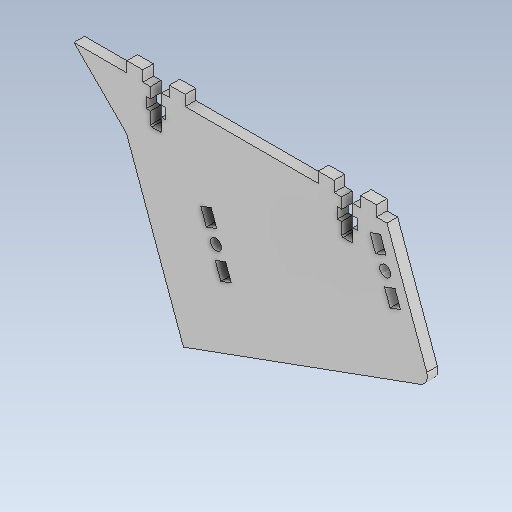
# Autodesk Inventor part: tc_support_front
Saved by Autodesk Inventor 2020.1 (Build 241239000, 239)
## iProperties
Created: 2019-07-16
Part Number: tc_support_front
Material: Acier inoxydable
Document SubType Name: Modeling
Designer: Thibault
Density: 8 g/cm^3
Appearance: Semi-poli
Author: Thibault
Autodesk Inventor part; units mm, degrees
ref_plane "YZ Plane" through (0, 0, 0) normal (1, 0, 0) x (0, 1, 0)
ref_plane "XZ Plane" through (0, 0, 0) normal (0, 1, 0) x (-1, 0, 0)
ref_plane "XY Plane" through (0, 0, 0) normal (0, 0, 1) x (1, 0, 0)
sketch "Anchor (screw side)" plane through (0, 0, 0) normal (0, 0, 1) x (1, 0, 0)
  circle A0 centre (93.7216, 50.3096) radius 1.05
  line L0 (91.2716, 51.3596) -> (88.1716, 51.3596)
  line L1 (88.1716, 51.3596) -> (88.1716, 49.2596)
  line L2 (88.1716, 49.2596) -> (91.2716, 49.2596)
  line L3 (91.2716, 49.2596) -> (91.2716, 51.3596)
  line L4 (99.2716, 51.3596) -> (96.1716, 51.3596)
  line L5 (96.1716, 51.3596) -> (96.1716, 49.2596)
  line L6 (96.1716, 49.2596) -> (99.2716, 49.2596)
  line L7 (99.2716, 49.2596) -> (99.2716, 51.3596)
  line L8 (91.2716, 51.3596) -> (96.1716, 49.2596) construction
  line L9 (96.1716, 51.3596) -> (91.2716, 49.2596) construction
  line L10 (86.1716, 53.3596) -> (101.2716, 53.3596) construction
  line L11 (101.2716, 53.3596) -> (101.2716, 47.2596) construction
  line L12 (101.2716, 47.2596) -> (86.1716, 47.2596) construction
  line L13 (86.1716, 47.2596) -> (86.1716, 53.3596) construction
  point P0 (103.5798, 50.1132)
  dimension "d27" = 2.1
  dimension "d28" = 3.1
  dimension "d29" = 2.1
  dimension "d32" = 4.9
  dimension "d34" = 2
  dimension "d35_1" = 2
  dimension "d36_1" = 2
  dimension "d37" = 2
  measures "d27" diameter of A0
  measures "d28" distance of L2.end L1.end
  measures "d29" distance of L1.end L0.end
  measures "d32" distance between parallel lines of L5 L3
  measures "d34" distance between parallel lines of L0 L10
  measures "d35_1" distance between parallel lines of L12 L2
  measures "d36_1" distance between parallel lines of L11 L7
  measures "d37" distance between parallel lines of L13 L1
sketch "Anchor (nut side)" plane through (0, 0, 0) normal (0, 0, 1) x (1, 0, 0)
  line L0 (10, 0) -> (8.55, 0)
  line L1 (8.55, 0) -> (8.55, -2)
  line L2 (8.55, -2) -> (9.35, -2)
  line L3 (9.35, -2) -> (9.35, -4)
  line L4 (5.65, -4) -> (5.65, -2)
  line L5 (5.65, -2) -> (6.45, -2)
  line L6 (6.45, -2) -> (6.45, 0)
  line L7 (6.45, 0) -> (5, 0)
  line L8 (2, 0) -> (2, 2)
  line L9 (2, 0) -> (3, 0) construction
  line L10 (2, 2) -> (5, 2)
  line L11 (5, 2) -> (5, 0)
  line L12 (10, 0) -> (10, 2)
  line L13 (10, 2) -> (13, 2)
  line L14 (13, 2) -> (13, 0)
  line L15 (0, 0) -> (2, 0)
  line L16 (13, 0) -> (15, 0)
  line L17 (5.65, -4) -> (6.45, -4)
  line L18 (9.35, -4) -> (8.55, -4)
  line L19 (6.45, -4) -> (6.45, -6.25)
  line L20 (8.55, -4) -> (8.55, -6.25)
  line L21 (6.7, -6.5) -> (7.5, -6.5)
  arc A0 (6.45, -6.25) -> (6.7, -6.5) centre (6.7, -6.25) ccw
  arc A1 (8.3, -6.5) -> (8.55, -6.25) centre (8.3, -6.25) ccw
  line L22 (7.5, -6.5) -> (8.3, -6.5)
  line L23 (7.5, -3.8983) -> (7.5, -9.959) construction
  point P0 (9.1321, -0.6227)
  point P1 (6.45, -6.5)
  point P2 (8.55, -6.5)
  dimension "d3" = 2
  dimension "d7" = 5
  dimension "d10" = 1.45
  dimension "d11" = 2
  dimension "d12" = 0.8
  dimension "d13" = 2
  dimension "d14" = 0.8
  dimension "d15" = 2.1
  dimension "d18" = 2
  dimension "d19" = 0.8
  dimension "d20" = 0.8
  dimension "d21" = 2.5
  dimension "d22" = 2.5
  dimension "d23" = 2.1
  dimension "d38" = 2
  dimension "d39" = 0.25
  dimension "d120" = 3
  measures "d3" distance of L15.start L8.start
  measures "d7" distance of L7.end L0.start
  measures "d10" distance of L0.start L0.end
  measures "d11" distance of L0.end L1.end
  measures "d12" distance of L1.end L2.end
  measures "d13" distance of L2.end L3.end
  measures "d14" distance of L4.end L5.end
  measures "d15" distance of L6.end L0.end
  measures "d18" distance of L14.end L16.end
  measures "d19" distance of L4.start L17.end
  measures "d20" distance of L3.end L18.end
  measures "d21" distance of L17.end point (6.45, -6.5)
  measures "d22" distance of L18.end point (8.55, -6.5)
  measures "d23" distance of L17.end L18.end
  measures "d38" distance between parallel lines of L15 L10
  measures "d39" radius of A0
  measures "d120" distance of L8.end L10.end
derived "shared_parameters.ipt"
sketch "Esquisse1" plane through (0, 0, 0) normal (0, 0, 1) x (1, 0, 0)
  line L0 (-13.2611, 6.6812) -> (7.8389, 6.6812)
  line L1 (-28.2611, 6.6812) -> (-36.2611, 6.6812)
  line L2 (-36.2611, 6.6812) -> (-26.3575, -3.2224)
  line L3 (30.3473, -13.9482) -> (22.8389, 6.6812)
  line L4 (29.152, -16.5116) -> (-15.5931, -32.7975)
  line L5 (-2.0657, -1.8526) -> (7.9343, -1.7975) construction
  arc A0 (29.152, -16.5116) -> (30.3473, -13.9482) centre (28.4679, -14.6322) ccw
  line L6 (-15.5931, -32.7975) -> (-26.3575, -3.2224)
  line L7 (-18.2611, 6.6812) -> (-19.7111, 6.6812)
  line L8 (-19.7111, 6.6812) -> (-19.7111, 4.6812)
  line L9 (-19.7111, 4.6812) -> (-18.9111, 4.6812)
  line L10 (-18.9111, 4.6812) -> (-18.9111, 2.6812)
  line L11 (-22.6111, 2.6812) -> (-22.6111, 4.6812)
  line L12 (-22.6111, 4.6812) -> (-21.8111, 4.6812)
  line L13 (-21.8111, 4.6812) -> (-21.8111, 6.6812)
  line L14 (-21.8111, 6.6812) -> (-23.2611, 6.6812)
  line L15 (-26.2611, 6.6812) -> (-26.2611, 8.6812)
  line L16 (-26.2611, 6.6812) -> (-25.2611, 6.6812) construction
  line L17 (-26.2611, 8.6812) -> (-23.2611, 8.6812)
  line L18 (-23.2611, 8.6812) -> (-23.2611, 6.6812)
  line L19 (-18.2611, 6.6812) -> (-18.2611, 8.6812)
  line L20 (-18.2611, 8.6812) -> (-15.2611, 8.6812)
  line L21 (-15.2611, 8.6812) -> (-15.2611, 6.6812)
  line L22 (-28.2611, 6.6812) -> (-26.2611, 6.6812)
  line L23 (-15.2611, 6.6812) -> (-13.2611, 6.6812)
  line L24 (-22.6111, 2.6812) -> (-21.8111, 2.6812)
  line L25 (-18.9111, 2.6812) -> (-19.7111, 2.6812)
  line L26 (-21.8111, 2.6812) -> (-21.8111, 0.4312)
  line L27 (-19.7111, 2.6812) -> (-19.7111, 0.4312)
  line L28 (-21.5611, 0.1812) -> (-20.7611, 0.1812)
  arc A1 (-21.8111, 0.4312) -> (-21.5611, 0.1812) centre (-21.5611, 0.4312) ccw
  arc A2 (-19.9611, 0.1812) -> (-19.7111, 0.4312) centre (-19.9611, 0.4312) ccw
  line L29 (-20.7611, 0.1812) -> (-19.9611, 0.1812)
  line L30 (-20.7611, 2.7829) -> (-20.7611, -3.2778) construction
  line L31 (17.8389, 6.6812) -> (16.3889, 6.6812)
  line L32 (16.3889, 6.6812) -> (16.3889, 4.6812)
  line L33 (16.3889, 4.6812) -> (17.1889, 4.6812)
  line L34 (17.1889, 4.6812) -> (17.1889, 2.6812)
  line L35 (13.4889, 2.6812) -> (13.4889, 4.6812)
  line L36 (13.4889, 4.6812) -> (14.2889, 4.6812)
  line L37 (14.2889, 4.6812) -> (14.2889, 6.6812)
  line L38 (14.2889, 6.6812) -> (12.8389, 6.6812)
  line L39 (9.8389, 6.6812) -> (9.8389, 8.6812)
  line L40 (9.8389, 6.6812) -> (10.8389, 6.6812) construction
  line L41 (9.8389, 8.6812) -> (12.8389, 8.6812)
  line L42 (12.8389, 8.6812) -> (12.8389, 6.6812)
  line L43 (17.8389, 6.6812) -> (17.8389, 8.6812)
  line L44 (17.8389, 8.6812) -> (20.8389, 8.6812)
  line L45 (20.8389, 8.6812) -> (20.8389, 6.6812)
  line L46 (7.8389, 6.6812) -> (9.8389, 6.6812)
  line L47 (20.8389, 6.6812) -> (22.8389, 6.6812)
  line L48 (13.4889, 2.6812) -> (14.2889, 2.6812)
  line L49 (17.1889, 2.6812) -> (16.3889, 2.6812)
  line L50 (14.2889, 2.6812) -> (14.2889, 0.4312)
  line L51 (16.3889, 2.6812) -> (16.3889, 0.4312)
  line L52 (14.5389, 0.1812) -> (15.3389, 0.1812)
  arc A3 (14.2889, 0.4312) -> (14.5389, 0.1812) centre (14.5389, 0.4312) ccw
  arc A4 (16.1389, 0.1812) -> (16.3889, 0.4312) centre (16.1389, 0.4312) ccw
  line L53 (15.3389, 0.1812) -> (16.1389, 0.1812)
  line L54 (15.3389, 2.7829) -> (15.3389, -3.2778) construction
  circle A5 centre (22.5049, -1.3188) radius 1.05
  line L55 (22.3561, -3.9802) -> (23.4164, -6.8932)
  line L56 (23.4164, -6.8932) -> (25.3898, -6.175)
  line L57 (25.3898, -6.175) -> (24.3295, -3.262)
  line L58 (24.3295, -3.262) -> (22.3561, -3.9802)
  line L59 (19.62, 3.5373) -> (20.6802, 0.6243)
  line L60 (20.6802, 0.6243) -> (22.6536, 1.3425)
  line L61 (22.6536, 1.3425) -> (21.5933, 4.2556)
  line L62 (21.5933, 4.2556) -> (19.62, 3.5373)
  line L63 (22.3561, -3.9802) -> (22.6536, 1.3425) construction
  line L64 (20.6802, 0.6243) -> (24.3295, -3.262) construction
  line L65 (22.2211, -9.4567) -> (17.0566, 4.7327) construction
  line L66 (17.0566, 4.7327) -> (22.7887, 6.819) construction
  line L67 (22.7887, 6.819) -> (27.9532, -7.3703) construction
  line L68 (27.9532, -7.3703) -> (22.2211, -9.4567) construction
  circle A6 centre (-9.4447, -12.9475) radius 1.05
  line L69 (-9.296, -10.2861) -> (-10.3562, -7.3731)
  line L70 (-10.3562, -7.3731) -> (-12.3296, -8.0913)
  line L71 (-12.3296, -8.0913) -> (-11.2693, -11.0044)
  line L72 (-11.2693, -11.0044) -> (-9.296, -10.2861)
  line L73 (-6.5598, -17.8037) -> (-7.6201, -14.8906)
  line L74 (-7.6201, -14.8906) -> (-9.5934, -15.6089)
  line L75 (-9.5934, -15.6089) -> (-8.5331, -18.5219)
  line L76 (-8.5331, -18.5219) -> (-6.5598, -17.8037)
  line L77 (-9.296, -10.2861) -> (-9.5934, -15.6089) construction
  line L78 (-7.6201, -14.8906) -> (-11.2693, -11.0044) construction
  line L79 (-9.1609, -4.8097) -> (-3.9964, -18.999) construction
  line L80 (-3.9964, -18.999) -> (-9.7285, -21.0854) construction
  line L81 (-9.7285, -21.0854) -> (-14.893, -6.896) construction
  line L82 (-14.893, -6.896) -> (-9.1609, -4.8097) construction
  point P0 (-13.2611, 6.6812)
  point P1 (31.0314, -15.8276)
  point P2 (22.4992, -2.0098)
  point P3 (22.5049, -1.3188)
  point P4 (-9.4447, -12.9475)
  dimension "d33" = 59.1
  dimension "d44" = 11
  dimension "d46" = 2
  dimension "d49" = 10
  dimension "d52" = 2
  dimension "d53" = 36
  dimension "d54" = 8
  dimension "d57" = 45
  dimension "d58" = 20
  constraints: 14 end point, 3 horizontal, 2 point on circle, 2 point on line, 2 tangent, 1 centre point, 1 parallel, 1 perpendicular, 6 other
  measures "d33" distance of L3.end L1.end
  measures "d46" radius of A0
  measures "d57" angle of L2 L1
  measures "d58" angle of L4 L0
extrude "Extrusion1" add sketch "Esquisse1" along normal blind 2
derived "tc_base_plate.ipt"
equation "\"d33\" = tc_base_width"
equation "\"d44\" = extra_height_front"
equation "\"d52\" = anchor_dist_a"
equation "\"d53\" = anchor_dist_b"
equation "\"d54\" = anchor_dist_top_a"
equation "\"d58\" = tilt_angle"
equation "\"d35\" = sheet_thickness"
equation "\"tc_base_width\" = 59.1"
equation "\"extra_height_front\" = 11"
equation "\"anchor_dist_a\" = 2"
equation "\"anchor_dist_b\" = 36"
equation "\"anchor_dist_top_a\" = 8"
equation "\"tilt_angle\" = 20deg"
equation "\"sheet_thickness\" = 2"
